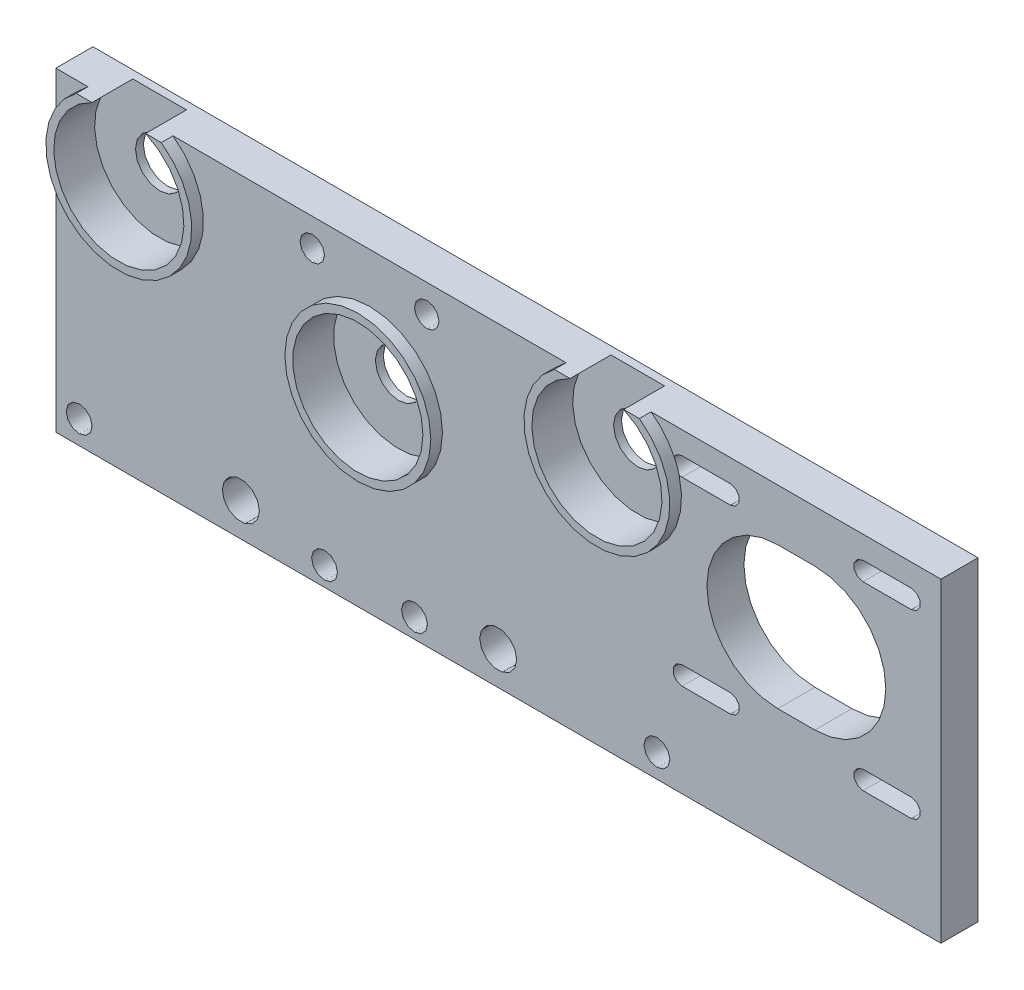
# Autodesk Inventor part: double-left2.0
Saved by Autodesk Inventor 2014 (Build 180170000, 170)
## iProperties
Created: 2013-11-04
Part Number: double-left2.0
Material: Generic
Document SubType Name: Modeling
Designer: stephen
Density: 1 g/cm^3
Appearance: Default
Author: stephen
Autodesk Inventor part; units mm, degrees
ref_plane "YZ Plane" through (0, 0, 0) normal (1, 0, 0) x (0, 1, 0)
ref_plane "XZ Plane" through (0, 0, 0) normal (0, 1, 0) x (-1, 0, 0)
ref_plane "XY Plane" through (0, 0, 0) normal (0, 0, 1) x (1, 0, 0)
sketch "Sketch1" plane through (0, 0, 0) normal (0, 0, 1) x (1, 0, 0)
  line L0 (187.5582, 20.5) -> (187.5582, 63.5)
  circle A0 centre (99.5007, 58.7375) radius 2.0955
  line L1 (174.2232, 59.6265) -> (182.4782, 59.6265)
  arc A1 (182.4782, 56.4515) -> (182.4782, 59.6265) centre (182.4782, 58.039) ccw
  line L2 (182.4782, 56.4515) -> (174.2232, 56.4515)
  arc A2 (174.2232, 59.6265) -> (174.2232, 56.4515) centre (174.2232, 58.039) ccw
  line L3 (143.2352, 59.6265) -> (151.4902, 59.6265)
  arc A3 (151.4902, 56.4515) -> (151.4902, 59.6265) centre (151.4902, 58.039) ccw
  line L4 (151.4902, 56.4515) -> (143.2352, 56.4515)
  arc A4 (143.2352, 59.6265) -> (143.2352, 56.4515) centre (143.2352, 58.039) ccw
  circle A5 centre (130.6347, 53.34) radius 4.15
  line L5 (143.2352, 28.6385) -> (151.4902, 28.6385)
  arc A6 (151.4902, 25.4635) -> (151.4902, 28.6385) centre (151.4902, 27.051) ccw
  line L6 (151.4902, 25.4635) -> (143.2352, 25.4635)
  arc A7 (143.2352, 28.6385) -> (143.2352, 25.4635) centre (143.2352, 27.051) ccw
  line L7 (174.2232, 28.6385) -> (182.4782, 28.6385)
  arc A8 (182.4782, 25.4635) -> (182.4782, 28.6385) centre (182.4782, 27.051) ccw
  line L8 (182.4782, 25.4635) -> (174.2232, 25.4635)
  arc A9 (174.2232, 28.6385) -> (174.2232, 25.4635) centre (174.2232, 27.051) ccw
  line L9 (187.5582, 63.5) -> (187.5582, 20.5)
  line L10 (89.6967, 42.545) -> (89.6967, 25.4635)
  circle A10 centre (48.7588, 53.34) radius 4.15
  circle A11 centre (79.8923, 58.737) radius 2.0955
  line L11 (35.9728, 63.5) -> (187.5582, 63.5)
  line L12 (187.5582, 63.5) -> (187.5582, 20.5)
  line L13 (35.9728, 63.5) -> (187.5582, 63.5)
  line L14 (187.5582, 63.5) -> (187.5582, 20.5)
  line L15 (187.5582, 63.5) -> (35.9728, 63.5)
  line L16 (187.5582, 20.5) -> (187.5582, 63.5)
  line L17 (35.9728, 63.5) -> (187.5582, 63.5)
  line L18 (187.5582, 63.5) -> (187.5582, 20.5)
  line L19 (187.5582, 20.5) -> (187.5582, 14.5)
  line L20 (35.9728, 14.5) -> (35.9728, 63.5)
  line L21 (38.7587, 53.34) -> (48.7587, 53.34)
  line L22 (84.6967, 42.545) -> (89.6967, 42.545)
  circle A12 centre (111.7312, 15.24) radius 3.175
  circle A13 centre (97.3962, 12.795) radius 2.2225
  circle A14 centre (81.9972, 12.795) radius 2.2225
  circle A15 centre (67.6622, 15.24) radius 3.175
  circle A16 centre (89.6967, 42.545) radius 4.15
  line L23 (67.6622, 15.24) -> (67.2997, 15.6892)
  line L24 (77.8053, 9.5347) -> (89.6967, 9.5347) construction
  line L25 (111.7312, 15.24) -> (118.0474, 15.24) construction
  line L26 (35.9728, 14.5) -> (35.9728, 9.5)
  line L27 (35.9728, 9.5) -> (187.5582, 9.5)
  line L28 (187.5582, 9.5) -> (187.5582, 14.5)
  circle A17 centre (67.6622, 15.24) radius 3.175
  circle A18 centre (81.9972, 12.795) radius 2.2225
  circle A19 centre (97.3962, 12.795) radius 2.2225
  circle A20 centre (111.7312, 15.24) radius 3.175
  line L29 (165.9682, 54.632) -> (159.6182, 54.632)
  arc A21 (159.6182, 54.632) -> (159.6182, 30.331) centre (159.6182, 42.4815) ccw
  line L30 (159.6182, 30.331) -> (165.9682, 30.331)
  arc A22 (165.9682, 30.331) -> (165.9682, 54.632) centre (165.9682, 42.4815) ccw
  line L31 (80.9972, 12.795) -> (81.9972, 12.795)
  line L32 (98.3962, 12.795) -> (97.3962, 12.795)
  line L33 (76.0442, 58.7375) -> (78.0442, 58.7375)
  line L34 (103.3492, 58.7375) -> (101.3492, 58.7375)
  line L35 (89.6967, 42.545) -> (89.6967, 65.1685)
  line L36 (101.3492, 58.7375) -> (89.6967, 58.7375)
  line L37 (89.6967, 58.7375) -> (79.8923, 58.7375)
  line L38 (165.9682, 42.4815) -> (165.9682, 63.5)
  line L39 (165.9682, 63.5) -> (187.5582, 63.5)
  point P0 (0, 0)
  point P1 (85.8435, 41.0037)
  point P2 (85.7775, 41.1803)
  point P3 (85.6109, 41.8173)
  point P4 (85.6694, 41.5431)
  point P5 (85.8646, 40.952)
  point P6 (85.8435, 44.0863)
  dimension "d4" = 8.3
  dimension "d55" = 10.16
  dimension "d56" = 10.16
  dimension "d57" = 4.7625
  dimension "d58" = 4.763
  dimension "d59" = 20.955
  dimension "d62" = 3.8735
  dimension "d63" = 27.813
  dimension "d66" = 3.8735
  dimension "d67" = 27.813
  dimension "d69" = 10
  dimension "d70" = 5
  dimension "d76" = 8.3
  dimension "d100" = 4.191
  dimension "d101" = 8.3
  dimension "d102" = 1
  dimension "d103" = 1
  dimension "d104" = 2
  dimension "d105" = 2
  dimension "d114" = 9.804
  dimension "d115" = 9.8044
  dimension "d120" = 9.8044
  constraints: 80 end point, 26 point on circle, 23 centre point, 9 perpendicular, 5 horizontal, 4 collinear, 4 concentric, 4 parallel, 2 coincident, 2 point on line
  measures "d4" diameter of A5
  measures "d55" distance from line of L13 A10.centre
  measures "d56" distance from line of L17 A5.centre
  measures "d57" distance from line of L17 A0.centre
  measures "d58" distance from line of L17 A11.centre
  measures "d59" distance from line of L17 L10.start
  measures "d62" distance between parallel lines of L11 L3
  measures "d63" distance between parallel lines of L5 L4
  measures "d66" distance between parallel lines of L17 L1
  measures "d67" distance between parallel lines of L7 L2
  measures "d69" distance of L21.start L21.end
  measures "d70" distance of L22.start L22.end
  measures "d76" diameter of A16
  measures "d100" diameter of A0
  measures "d101" diameter of A10
  measures "d102" distance of L31.start L31.end
  measures "d103" distance of L32.start L32.end
  measures "d104" distance of L33.start L33.end
  measures "d105" distance of L34.start L34.end
  measures "d114" distance from line of A0.centre L35
  measures "d115" distance of L36.end L37.end
  measures "d120" distance from line of L35 L37.end
ref_plane "Work Plane6" through (0, 0, 6.35) normal (0, 0, 1) x (1, 0, 0)
extrude "Extrusion18" add sketch "Sketch1" along normal blind 6.35 contours L19 L28 L27 L26 L20 L11 L0 | L35 A16 L10 | L10 A16 L22 | L22 A16 L35 | A22 L30 A21 L29
ref_plane "Work Plane11" through (0, 0, 6.35) normal (0, 0, 1) x (1, 0, 0)
sketch "Sketch9" plane through (0, 0, 6.35) normal (0, 0, 1) x (1, 0, 0)
  circle A0 centre (48.7588, 53.34) radius 4 projected
  line L0 (187.5582, 63.5) -> (25.9728, 63.5) projected
  arc A1 (44.1657, 63.5) -> (53.3519, 63.5) centre (48.7588, 53.34) ccw
  arc A2 (41.477, 63.5) -> (56.0406, 63.5) centre (48.7588, 53.34) ccw
  point P0 (0, 0)
  dimension "d32" = 22.3
  dimension "d33" = 25
  constraints: 4 point on circle, 4 point on line, 2 centre point, 2 coincident
  measures "d32" diameter of A1
  measures "d33" diameter of A2
extrude "Extrusion10" add sketch "Sketch9" along normal blind 2 contours A2 L0 A1
ref_plane "Work Plane10" through (0, 0, 6.35) normal (0, 0, 1) x (1, 0, 0)
ref_plane "Work Plane9" through (0, 0, 6.35) normal (0, 0, 1) x (1, 0, 0)
sketch "Sketch11" plane through (0, 0, 6.35) normal (0, 0, 1) x (1, 0, 0)
  circle A0 centre (89.6967, 42.545) radius 4 projected
  circle A1 centre (89.6967, 42.545) radius 11.15
  circle A2 centre (89.6967, 42.545) radius 12.5
  point P0 (0, 0)
  dimension "d40" = 22.3
  dimension "d41" = 25
  constraints: 2 centre point, 2 coincident
  measures "d40" diameter of A1
  measures "d41" diameter of A2
extrude "Extrusion12" add sketch "Sketch11" along normal blind 2 contours A2
ref_plane "Work Plane7" through (0, 0, 6.35) normal (0, 0, 1) x (1, 0, 0)
ref_plane "Work Plane8" through (0, 0, 6.35) normal (0, 0, 1) x (1, 0, 0)
ref_plane "Work Plane12" through (89.6967, 42.545, 6.35) normal (0, 0, 1) x (1, 0, 0)
sketch "Sketch15" plane through (89.6967, 42.545, 6.35) normal (0, 0, 1) x (1, 0, 0)
  circle A0 centre (0, 0) radius 11.15 projected
  circle A1 centre (0, 0) radius 4 projected
  point P0 (-89.6967, -42.545)
sketch "Sketch17" plane through (0, 0, 6.35) normal (0, 0, 1) x (1, 0, 0)
  arc A0 (44.1657, 63.5) -> (53.3519, 63.5) centre (48.7588, 53.34) ccw projected
  line L0 (53.3519, 63.5) -> (44.1657, 63.5) projected
  circle A1 centre (48.7588, 53.34) radius 4.15 projected
  point P0 (0, 0)
extrude "Extrusion22" cut sketch "Sketch17" against normal blind 5
sketch "Sketch10" plane through (0, 0, 6.35) normal (0, 0, 1) x (1, 0, 0)
  line L0 (52.9748, 63.5) -> (56.0406, 63.5) projected
  circle A0 centre (130.6347, 53.34) radius 4 projected
  arc A1 (126.0415, 63.5) -> (135.2278, 63.5) centre (130.6347, 53.34) ccw
  arc A2 (123.3529, 63.5) -> (137.9164, 63.5) centre (130.6347, 53.34) ccw
  line L1 (187.5582, 63.5) -> (56.0406, 63.5) projected
  line L2 (123.3529, 63.5) -> (126.0415, 63.5)
  line L3 (135.2278, 63.5) -> (137.9164, 63.5)
  arc A3 (126.0415, 63.5) -> (135.2278, 63.5) centre (130.6347, 53.34) ccw
  arc A4 (123.3529, 63.5) -> (137.9164, 63.5) centre (130.6347, 53.34) ccw
  line L4 (123.3529, 63.5) -> (137.9164, 63.5)
  point P0 (0, 0)
  dimension "d82" = 11.15
  constraints: 8 point on circle, 6 end point, 4 centre point, 4 coincident, 4 point on line, 3 collinear, 2 concentric
  measures "d82" radius of A1
extrude "Extrusion26" cut sketch "Sketch10" against normal blind 5 contours L1 A1
sketch "Sketch21" plane through (0, 0, 6.35) normal (0, 0, 1) x (1, 0, 0)
  arc A0 (126.0415, 63.5) -> (135.2278, 63.5) centre (130.6347, 53.34) ccw projected
  line L0 (126.0415, 63.5) -> (56.0406, 63.5) projected
  line L1 (187.5582, 63.5) -> (135.2278, 63.5) projected
  arc A1 (123.3529, 63.5) -> (137.9164, 63.5) centre (130.6347, 53.34) ccw
  line L2 (123.3529, 63.5) -> (126.0415, 63.5)
  line L3 (135.2278, 63.5) -> (137.9164, 63.5)
  point P0 (0, 0)
  dimension "d97" = 25
  constraints: 4 end point, 4 point on circle, 2 point on line, 1 centre point, 1 coincident
  measures "d97" diameter of A1
extrude "Extrusion27" add sketch "Sketch21" along normal blind 2
sketch "Sketch22" plane through (0, 0, 6.35) normal (0, 0, 1) x (1, 0, 0)
  line L0 (35.9728, 63.5) -> (35.9728, 9.5) projected
  line L1 (35.9728, 9.5) -> (187.5582, 9.5) projected
  circle A0 centre (39.9728, 13.5) radius 2.2225
  point P0 (0, 0)
  dimension "d106" = 4
  dimension "d107" = 4
  constraints: 1 centre point
  measures "d106" distance from line of A0.centre L1
  measures "d107" distance from line of L0 A0.centre
extrude "Extrusion28" cut sketch "Sketch22" against normal through all
sketch "Sketch23" plane through (0, 0, 6.35) normal (0, 0, 1) x (1, 0, 0)
  circle A0 centre (39.9728, 13.5) radius 2.2225 projected
  line L0 (35.9728, 9.5) -> (187.5582, 9.5) projected
  circle A1 centre (138.9208, 13.5) radius 2.2225
  point P0 (0, 0)
  dimension "d110" = 4
  dimension "d111" = 98.948
  constraints: 1 centre point
  measures "d110" distance from line of L0 A1.centre
  measures "d111" distance of A1.centre A0.centre
extrude "Extrusion29" cut sketch "Sketch23" against normal through all contours A1
extrude "Extrusion30" cut sketch "Sketch15" against normal blind 5
sketch "Sketch24" plane through (89.6967, 42.545, 6.35) normal (0, 0, 1) x (1, 0, 0)
  circle A0 centre (0, 0) radius 4 projected
  point P0 (-89.6967, -42.545)
extrude "Extrusion31" cut sketch "Sketch24" against normal through all
sketch "Sketch25" plane through (0, 0, 6.35) normal (0, 0, 1) x (1, 0, 0)
  line L0 (165.9682, 54.632) -> (159.6182, 54.632)
  arc A0 (159.6182, 54.632) -> (159.6182, 30.331) centre (159.6182, 42.4815) ccw
  line L1 (159.6182, 30.331) -> (165.9682, 30.331)
  arc A1 (165.9682, 30.331) -> (165.9682, 54.632) centre (165.9682, 42.4815) ccw
  line L2 (165.9682, 42.4815) -> (165.9682, 63.5)
  line L3 (165.9682, 63.5) -> (187.5582, 63.5)
  point P0 (0, 0)
  constraints: 8 end point, 4 point on circle, 2 centre point
extrude "Extrusion32" cut sketch "Sketch25" against normal through all
body "Solid2"
